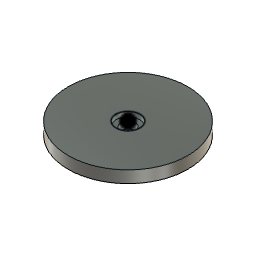
_Paper roll arm _ grip arm cap.a85ccca9-b7a4-4d6e-98ef-0463d6195870 (Autodesk Fusion 360 design; units mm, degrees)
Autodesk Fusion 360 part; units mm, degrees
sketch "Sketch1" plane through (0, 0, 0) normal (0, 0, 1) x (1, 0, 0)
  circle A0 centre (0, 0) radius 25
  dimension "d1" = 50
  constraint coincident A0.centre origin
  measures "d1" diameter of A0
extrude "Extrude1" add sketch "Sketch1" along normal blind 5
sketch "Sketch2" plane through (0, 0, 5) normal (0, 0, 1) x (-1, 0, 0)
  circle A0 centre (0, 0) radius 25
  circle A1 centre (0, 0) radius 5
  dimension "d4" = 10
  constraint coincident A0.centre A1.centre
  measures "d4" diameter of A1
extrude "Extrude3" cut sketch "Sketch2" against normal blind 2 contours A1
sketch "Sketch3" plane through (0, 0, 5) normal (0, 0, 1) x (-1, 0, 0)
  circle A0 centre (0, 0) radius 3
  dimension "d9" = 6
  constraint coincident A0.centre origin
  measures "d9" diameter of A0
extrude "Extrude4" cut sketch "Sketch3" against normal blind 5
